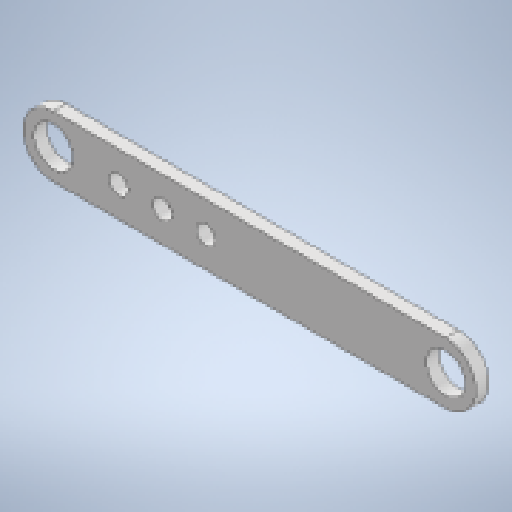
# Autodesk Inventor part: free_link
Saved by Autodesk Inventor 2025.1 (Build 291241000, 241)
## iProperties
Created: 2024-09-02
Part Number: free_link
Material: 一般
Document SubType Name: Modeling
Designer: right
Density: 1 g/cm^3
Appearance: 既定
Author: right
Autodesk Inventor part; units mm, degrees
ref_plane "YZ Plane" through (0, 0, 0) normal (1, 0, 0) x (0, 1, 0)
ref_plane "XZ Plane" through (0, 0, 0) normal (0, 1, 0) x (-1, 0, 0)
ref_plane "XY Plane" through (0, 0, 0) normal (0, 0, 1) x (1, 0, 0)
sketch "スケッチ1" plane through (0, 0, 0) normal (0, 0, 1) x (1, 0, 0)
  line L0 (-22.5, -3.5) -> (22.5, -3.5)
  line L1 (22.5, -3.5) -> (22.5, 3.5) construction
  line L2 (22.5, 3.5) -> (-22.5, 3.5)
  line L3 (-22.5, 3.5) -> (-22.5, -3.5) construction
  line L4 (-22.5, -3.5) -> (22.5, 3.5) construction
  line L5 (22.5, -3.5) -> (-22.5, 3.5) construction
  circle A0 centre (-22.5, 0) radius 3.5
  line L6 (0, 3.5) -> (0, -3.5) construction
  circle A1 centre (22.5, 0) radius 3.5
  circle A2 centre (-22.5, 0) radius 2.25
  circle A3 centre (22.5, 0) radius 2.25
  point P0 (0, 0)
  point P1 (22.5, -3.5)
  point P2 (22.5, 3.5)
  dimension "d0" = 7
  dimension "d1" = 45
  dimension "d2" = 4.5
  constraints: 14 end point, 5 midpoint, 3 centre point, 2 parallel, 2 symmetric about line, 1 coincident, 1 horizontal, 1 perpendicular, 5 other
  measures "d1" distance of L1.end L2.end
  measures "d2" diameter of A2
extrude "押し出し1" add sketch "スケッチ1" along normal blind 1.5
sketch "スケッチ2" plane through (0, 0, 1.5) normal (0, 0, 1) x (1, 0, 0)
  circle A0 centre (22.5, 0) radius 2.25 construction
  circle A1 centre (-22.5, 0) radius 2.25 construction
  line L0 (22.5, 0) -> (-22.5, 0) construction
  circle A2 centre (0, 0) radius 1.1
  circle A3 centre (-5, 0) radius 1.1
  circle A4 centre (-10, 0) radius 1.1
  circle A5 centre (-15, 0) radius 1.1
  circle A6 centre (-20, 0) radius 1.1
  circle A7 centre (5, 0) radius 1.1
  circle A8 centre (0, 0) radius 1.1
  circle A9 centre (-5, 0) radius 1.1
  circle A10 centre (-10, 0) radius 1.1
  circle A11 centre (-15, 0) radius 1.1
  circle A12 centre (10, 0) radius 1.1
  circle A13 centre (5, 0) radius 1.1
  circle A14 centre (0, 0) radius 1.1
  circle A15 centre (-5, 0) radius 1.1
  circle A16 centre (-10, 0) radius 1.1
  circle A17 centre (15, 0) radius 1.1
  circle A18 centre (10, 0) radius 1.1
  circle A19 centre (5, 0) radius 1.1
  circle A20 centre (0, 0) radius 1.1
  circle A21 centre (-5, 0) radius 1.1
  circle A22 centre (20, 0) radius 1.1
  circle A23 centre (15, 0) radius 1.1
  circle A24 centre (10, 0) radius 1.1
  circle A25 centre (5, 0) radius 1.1
  circle A26 centre (0, 0) radius 1.1
  dimension "d5" = 2.2
  dimension "d8" = 5
  dimension "d11" = 5
  constraints: 25 centre point, 3 horizontal, 2 end point, 1 coincident, 48 other
  measures "d5" diameter of A2
  measures "d8" distance of A2.centre A3.centre
  measures "d11" distance of A2.centre A7.centre
extrude "押し出し2" cut sketch "スケッチ2" against normal through all contours A2 | A3 | A7
